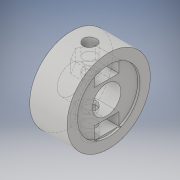
# Autodesk Inventor part: Swivel Joint Axle Lock Grub Screw
Saved by Autodesk Inventor 2019 (Build 230136000, 136)
## iProperties
Created: 2020-04-05
Part Number: Swivel Joint Axle Lock Grub Screw
Material: Generic
Document SubType Name: Modeling
Designer: isaac
Density: 1 g/cm^3
Appearance: Default
Author: isaac
Autodesk Inventor part; units mm, degrees
ref_plane "YZ Plane" through (0, 0, 0) normal (1, 0, 0) x (0, 1, 0)
ref_plane "XY Plane" through (0, 0, 0) normal (0, 0, 1) x (1, 0, 0)
sketch "Sketch9" plane through (0, 0, 0) normal (1, 0, 0) x (0, 1, 0)
  circle A0 centre (0, 0) radius 10
  circle A1 centre (0, 0) radius 3.4
  dimension "d31" = 20
  dimension "d32" = 6.8
  constraints: 2 centre point, 2 coincident
  measures "d31" diameter of A0
  measures "d32" diameter of A1
extrude "Extrusion7" add sketch "Sketch9" along normal blind 9
sketch "Sketch10" plane through (9, 0, 0) normal (1, 0, 0) x (0, 0, -1)
  circle A0 centre (0, 0) radius 7.5
  dimension "d35" = 15
  constraints: 1 centre point, 1 coincident
  measures "d35" diameter of A0
extrude "Extrusion8" cut sketch "Sketch10" against normal blind 0.5
ref_plane "Work Plane3" through (0, 5.5, 0) normal (0, 1, 0) x (-1, 0, 0)
sketch "Sketch11" plane through (0, 5.5, 0) normal (0, 1, 0) x (-1, 0, 0)
  line L0 (0, 0) -> (-9, 0) construction
  line L1 (-9, 10) -> (-9, -10) construction
  line L2 (-7.9064, 0) -> (-6.2032, 2.95)
  line L3 (-6.2032, 2.95) -> (-2.7968, 2.95)
  line L4 (-2.7968, 2.95) -> (-1.0936, 0)
  line L5 (-1.0936, 0) -> (-2.7968, -2.95)
  line L6 (-2.7968, -2.95) -> (-6.2032, -2.95)
  line L7 (-6.2032, -2.95) -> (-7.9064, 0)
  line L8 (-6.2032, 2.95) -> (-9, 2.95)
  line L9 (-9, 2.95) -> (-9, -2.95)
  line L10 (-9, -2.95) -> (-6.2032, -2.95)
  point P0 (-4.5, 0)
  dimension "d39" = 5.9
  constraints: 20 end point, 3 point on line, 2 midpoint, 1 horizontal, 1 perpendicular, 13 other
  measures "d39" distance between parallel lines of L6 L3
extrude "Extrusion9" cut sketch "Sketch11" along normal mid plane 3
ref_plane "Work Plane4" through (0, 10, 0) normal (0, 1, 0) x (-1, 0, 0)
sketch "Sketch12" plane through (0, 10, 0) normal (0, 1, 0) x (-1, 0, 0)
  line L0 (-2.7968, 2.95) -> (-1.0936, 0) construction
  line L1 (-1.9452, 1.475) -> (-5.8393, -0.7732) construction
  line L2 (-1.0936, 0) -> (-2.7968, -2.95) construction
  line L3 (-1.9452, -1.475) -> (-5.6209, 0.6472) construction
  circle A0 centre (-4.5, 0) radius 2.95 construction
  point P0 (0, 0)
  constraints: 4 end point, 2 midpoint, 2 perpendicular, 2 point on line, 1 coincident, 3 other
hole "Hole2" at (4.5, 10, 0) direction (0, -1, 0) diameter 3.1 depth 10
mirror "Mirror2" about plane through (0, 0, 0) normal (0, 1, 0) of "Extrusion9", "Hole2"
body "Solid2"
